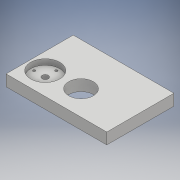
# Autodesk Inventor part: Flancs
Saved by Autodesk Inventor 2017 SP1 (Build 210196100, 196)
## iProperties
Part Number: Flancs
Material: Générique
Document SubType Name: Modeling
Designer: Sylvain
Density: 1 g/cm^3
Appearance: Par défaut
Author: Sylvain
Autodesk Inventor part; units mm, degrees
ref_plane "YZ Plane" through (0, 0, 0) normal (1, 0, 0) x (0, 1, 0)
ref_plane "XZ Plane" through (0, 0, 0) normal (0, 1, 0) x (-1, 0, 0)
ref_plane "XY Plane" through (0, 0, 0) normal (0, 0, 1) x (1, 0, 0)
sketch "Esquisse1" plane through (0, 0, 0) normal (0, 0, 1) x (1, 0, 0)
  line L0 (0, 0) -> (90, 0)
  line L1 (90, 0) -> (90, 60)
  line L2 (90, 60) -> (0, 60)
  line L3 (0, 60) -> (0, 0)
  dimension "d0" = 90
  dimension "d1" = 60
  constraints: 8 end point, 2 parallel, 1 horizontal, 1 perpendicular
  measures "d0" distance of L1.end L2.end
  measures "d1" distance of L0.end L1.end
extrude "Extrusion1" add sketch "Esquisse1" along normal blind 10
sketch "Esquisse2" plane through (0, 0, 10) normal (0, 0, 1) x (1, 0, 0)
  circle A0 centre (15, 20) radius 13
  line L0 (0, 0) -> (90, 0) projected
  line L1 (0, 60) -> (0, 0) projected
  circle A1 centre (75, 15) radius 13
  line L2 (90, 0) -> (90, 60) projected
  circle A2 centre (15, 29.9) radius 1.1
  circle A3 centre (5.1, 20) radius 1.1
  circle A4 centre (15, 10.1) radius 1.1
  circle A5 centre (24.9, 20) radius 1.1
  circle A6 centre (15, 20) radius 2.75
  dimension "d4" = 26
  dimension "d5" = 20
  dimension "d6" = 15
  dimension "d7" = 26
  dimension "d8" = 15
  dimension "d9" = 15
  dimension "d10" = 2.2
  dimension "d11" = 2
  dimension "d12" = 15
  dimension "d15" = 360
  dimension "d17" = 5.5
  constraints: 7 centre point, 1 coincident, 9 other
  measures "d4" diameter of A0
  measures "d5" distance from line of L0 A0.centre
  measures "d6" distance from line of L1 A0.centre
  measures "d7" diameter of A1
  measures "d8" distance from line of L0 A1.centre
  measures "d9" distance from line of L2 A1.centre
  measures "d10" diameter of A2
  measures "d12" distance from line of L1 A2.centre
  measures "d17" diameter of A6
extrude "Extrusion2" cut sketch "Esquisse2" against normal blind 10 contours A2 | A3 | A4 | A5 | A6
sketch "Esquisse3" plane through (0, 0, 10) normal (0, 0, 1) x (1, 0, 0)
  circle A0 centre (45, 22) radius 11
  line L0 (0, 0) -> (90, 0) projected
  line L1 (90, 0) -> (90, 60) projected
  dimension "d20" = 22
  dimension "d21" = 45
  dimension "d22" = 22
  constraints: 1 centre point
  measures "d20" distance from line of L0 A0.centre
  measures "d21" distance from line of L1 A0.centre
  measures "d22" diameter of A0
extrude "Extrusion3" cut sketch "Esquisse3" against normal blind 10
sketch "Esquisse4" plane through (0, 0, 10) normal (0, 0, 1) x (1, 0, 0)
  circle A0 centre (15, 20) radius 2.75 projected
  circle A1 centre (15, 20) radius 13
  point P0 (0, 0)
  dimension "d25" = 26
  constraints: 1 centre point, 1 coincident
  measures "d25" diameter of A1
extrude "Extrusion4" cut sketch "Esquisse4" against normal blind 5
